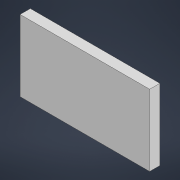
# Autodesk Inventor part: Деталь7
Saved by Autodesk Inventor 2022 (Build 260153070, 153G)
## iProperties
Created: 2021-12-15
Part Number: Деталь7
Material: Типовые
Document SubType Name: Sheet Metal
Designer: kalugin_a
Density: 1 g/cm^3
Flat Pattern Width: 1.04544 cm
Flat Pattern Length: 1.90161 cm
Flat Pattern Area: 1.98803 cm^2
Sheet Metal Rule: По умолчанию
Sheet Metal Width: 10,454 мм
Sheet Metal Length: 19,016 мм
Sheet Metal Area: 198,803 мм^2
Appearance: По умолчанию
Author: kalugin_a
Autodesk Inventor part; units mm, degrees
ref_plane "YZ Plane" through (0, 0, 0) normal (1, 0, 0) x (0, 1, 0)
ref_plane "XZ Plane" through (0, 0, 0) normal (0, 1, 0) x (-1, 0, 0)
ref_plane "XY Plane" through (0, 0, 0) normal (0, 0, 1) x (1, 0, 0)
sketch "Эскиз1" plane through (0, 0, 0) normal (0, 0, 1) x (1, 0, 0)
  line L0 (0, 0) -> (19.0161, 0)
  line L1 (19.0161, 0) -> (19.0161, 10.4544)
  line L2 (19.0161, 10.4544) -> (0, 10.4544)
  line L3 (0, 10.4544) -> (0, 0)
extrude "Пластина1" add sketch "Эскиз1" along normal blind 1.5
equation "\"d0\" = Толщина"
equation "\"Радиус_гибки\" = Толщина"
equation "\"Ширина_просечки\" = Толщина"
equation "\"Глубина_просечки\" = 0.5 * Толщина"
equation "\"Размер_просечки\" = 4 * Толщина"
equation "\"Мин_остаток\" = 2 * Толщина"
equation "\"Радиус_перехода\" = Радиус_гибки"
equation "\"Радиус_Якоби\" = Радиус_гибки"
equation "\"Размер_зазора\" = Толщина"
equation "\"Толщина\" = 1.5"
